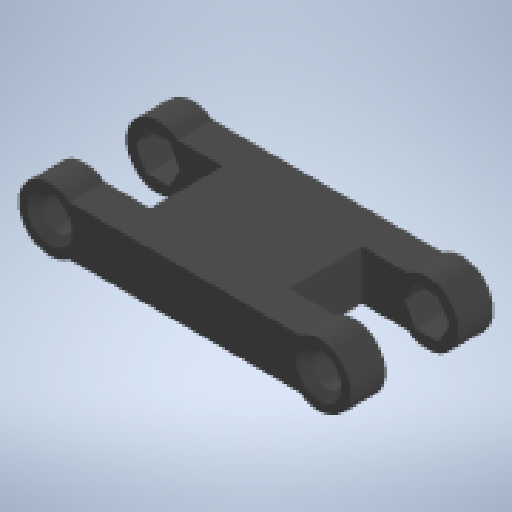
# Autodesk Inventor part: Barra1_0001_001
Saved by Autodesk Inventor 2025.2 (Build 292293000, 293)
## iProperties
Created: 2025-05-22
Part Number: Barra1_0001_001
Material: Borracha
Document SubType Name: Modeling
Designer: Gustavo Sousa
Density: 0.93 g/cm^3
Appearance: Borracha - Preta
Author: Gustavo Sousa
Autodesk Inventor part; units mm, degrees
ref_plane "YZ Plane" through (0, 0, 0) normal (1, 0, 0) x (0, 1, 0)
ref_plane "XZ Plane" through (0, 0, 0) normal (0, 1, 0) x (-1, 0, 0)
ref_plane "XY Plane" through (0, 0, 0) normal (0, 0, 1) x (1, 0, 0)
sketch "Esboço1" plane through (0, 0, 0) normal (0, 0, 1) x (1, 0, 0)
  line L0 (-12.7424, 2.75) -> (12.7424, 2.75)
  line L1 (-12.7424, -2.75) -> (12.7424, -2.75)
  circle A0 centre (-14.9075, 0) radius 3.5
  circle A1 centre (14.9075, 0) radius 3.5
  circle A2 centre (-14.9075, 0) radius 2.5
  circle A3 centre (14.9075, 0) radius 2.5
  point P0 (0, 0)
  point P1 (0, 2.75)
  point P2 (0, -2.75)
  dimension "d7" = 7
  dimension "d5" = 2.75
  dimension "d6" = 2.75
  dimension "d9" = 14.9075
  dimension "d11" = 29.815
  dimension "d12" = 5
  dimension "d13" = 5
  constraints: 4 end point, 3 centre point, 2 coincident, 2 horizontal, 2 horizontal alignment, 2 midpoint, 2 vertical alignment, 1 parallel, 4 other
  measures "d5" distance of point (0, 0) point (0, 2.75)
  measures "d6" distance of point (0, 0) point (0, -2.75)
  measures "d9" distance of point (0, 0) point (-14.908, 0)
  measures "d11" distance of point (-14.908, 0) A1.centre
  measures "d12" diameter of A2
  measures "d13" diameter of A3
extrude "Extrusão1" add sketch "Esboço1" along normal mid plane 3.9 contours L0 A1 L1 A0 | A0 | A1 | A2 | A3
sketch "Esboço2" plane through (0, 0, -1.95) normal (0, 0, -1) x (-1, 0, 0)
  line L0 (-7.7154, -2.75) -> (7.7154, -2.75)
  line L1 (7.7154, -2.75) -> (7.7154, 2.75)
  line L2 (7.7154, 2.75) -> (-7.7154, 2.75)
  line L3 (-7.7154, 2.75) -> (-7.7154, -2.75)
  line L4 (-7.7154, -2.75) -> (7.7154, 2.75) construction
  line L5 (7.7154, -2.75) -> (-7.7154, 2.75) construction
  line L6 (12.7424, 2.75) -> (-12.7424, 2.75) projected
  line L7 (-12.7424, -2.75) -> (12.7424, -2.75) projected
  point P0 (0, 0)
  point P1 (0, 2.75)
  point P2 (0, -2.75)
  point P3 (7.7154, 0)
  point P4 (0, 2.75)
  dimension "d21" = 15.4307
  constraints: 12 end point, 8 midpoint, 1 horizontal, 1 horizontal alignment, 1 parallel, 1 perpendicular, 1 vertical alignment
  measures "d21" distance of L1.end L2.end
extrude "Extrusão2" add sketch "Esboço2" along normal blind 8.04
sketch "Esboço3" plane through (0, 0, 1.95) normal (0, 0, 1) x (1, 0, 0)
  arc A0 (12.7424, -2.75) -> (12.7424, 2.75) centre (14.9075, 0) ccw projected
  point P0 (0, 0)
  constraints: 1 coincident
hole "Furo1" at (14.9075, 0, 1.95) direction (0, 0, -1) diameter 3.5 end through all countersink diameter 5 countersink angle 82
sketch "Esboço4" plane through (0, 0, 1.95) normal (0, 0, 1) x (1, 0, 0)
  arc A0 (-12.7424, 2.75) -> (-12.7424, -2.75) centre (-14.9075, 0) ccw projected
  point P0 (0, 0)
  constraints: 1 coincident
hole "Furo2" at (-14.9075, 0, 1.95) direction (0, 0, -1) diameter 3.5 end through all countersink diameter 5 countersink angle 82
sketch "Esboço5" plane through (0, 0, -9.99) normal (0, 0, -1) x (-1, 0, 0)
  arc A0 (-12.7424, 2.75) -> (-12.7424, -2.75) centre (-14.9075, 0) ccw projected
  circle A1 centre (-14.9075, 0) radius 3.5
  arc A2 (12.7424, -2.75) -> (12.7424, 2.75) centre (14.9075, 0) ccw projected
  circle A3 centre (14.9075, 0) radius 3.5
  line L0 (-12.7424, 2.75) -> (12.7424, 2.75)
  line L1 (-12.7424, -2.75) -> (12.7424, -2.75)
  circle A4 centre (-14.9075, 0) radius 2.5 projected
  line L2 (-13.6575, -2.1651) -> (-16.1575, -2.1651)
  line L3 (-16.1575, -2.1651) -> (-17.4075, 0)
  line L4 (-17.4075, 0) -> (-16.1575, 2.1651)
  line L5 (-16.1575, 2.1651) -> (-13.6575, 2.1651)
  line L6 (-13.6575, 2.1651) -> (-12.4075, 0)
  line L7 (-12.4075, 0) -> (-13.6575, -2.1651)
  circle A5 centre (14.9075, 0) radius 2.5 projected
  line L8 (13.6575, -2.1651) -> (12.4075, 0)
  line L9 (12.4075, 0) -> (13.6575, 2.1651)
  line L10 (13.6575, 2.1651) -> (16.1575, 2.1651)
  line L11 (16.1575, 2.1651) -> (17.4075, 0)
  line L12 (17.4075, 0) -> (16.1575, -2.1651)
  line L13 (16.1575, -2.1651) -> (13.6575, -2.1651)
  point P0 (0, 0)
  point P1 (-12.7424, -2.75)
  point P2 (-12.7424, 2.75)
  dimension "d37" = 7
  constraints: 28 end point, 4 coincident, 2 horizontal alignment, 1 centre point, 1 horizontal, 33 other
  measures "d37" diameter of A1
extrude "Extrusão3" add sketch "Esboço5" along normal blind 3.9 contours A1 A0 | L0 A3 L1 A1 | A2 A3 | L6 A4 | A4 L7 | L5 A4 | A4 L2 | L4 A4 | A4 L3 | L11 A5 | A5 L12 | L10 A5 | A5 L13 | L9 A5 | A5 L8
equation "\"d6\" = d5"
